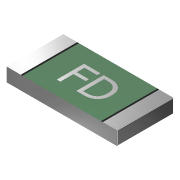
# Autodesk Inventor part: fuse
Saved by Autodesk Inventor 2012 (Build 160160000, 160)
## iProperties
Created: 2015-04-13
Part Number: fuse
Material: Default
Document SubType Name: Modeling
Designer: s42851
Density: 1 g/cm^3
Author: s42851
Autodesk Inventor part; units mm, degrees
ref_plane "YZ Plane" through (0, 0, 0) normal (1, 0, 0) x (0, 1, 0)
ref_plane "XZ Plane" through (0, 0, 0) normal (0, 1, 0) x (-1, 0, 0)
ref_plane "XY Plane" through (0, 0, 0) normal (0, 0, 1) x (1, 0, 0)
sketch "Sketch1" plane through (0, 0, 0) normal (0, 0, 1) x (1, 0, 0)
  line L0 (0, 0) -> (3.25, 0)
  line L1 (3.25, 0) -> (3.25, 1.65)
  line L2 (3.25, 1.65) -> (0, 1.65)
  line L3 (0, 1.65) -> (0, 0)
  dimension "d0" = 1.65
  dimension "d1" = 3.25
  constraints: 8 end point, 2 parallel, 1 horizontal, 1 perpendicular
  measures "d0" distance of L2.end L0.start
  measures "d1" distance of L0.start L0.end
extrude "Extrusion1" add sketch "Sketch1" along normal blind 0.4
sketch "Sketch2" plane through (0, 0, 0.4) normal (0, 0, 1) x (1, 0, 0)
  line L0 (0, 0) -> (0, 1.65) projected
  line L1 (3.25, 0) -> (0, 0) projected
  line L2 (0, 1.65) -> (3.25, 1.65) projected
  line L3 (0.425, 1.65) -> (0.425, 0)
  line L4 (0.475, 1.65) -> (0.475, 0)
  line L5 (0.425, 1.65) -> (0.475, 1.65)
  line L6 (0.425, 0) -> (0.475, 0)
  dimension "d4" = 0.425
  dimension "d7" = 0.05
  constraints: 8 end point, 2 parallel, 2 point on line, 1 collinear, 1 perpendicular
  measures "d4" distance between parallel lines of L0 L3
  measures "d7" distance between parallel lines of L3 L4
extrude "Extrusion2" cut sketch "Sketch2" against normal blind 0.001 contours L3 L2 L4 L1
ref_plane "Work Plane1" through (1.625, 0, 0) normal (1, 0, 0) x (0, 0, -1)
mirror "Mirror1" about plane through (1.625, 0, 0) normal (1, 0, 0) of "Extrusion2"
sketch "Sketch3" plane through (0, 0, 0.4) normal (0, 0, 1) x (1, 0, 0)
  line L0 (0.9936, 1.2023) -> (2.3385, 1.2023) construction
  line L1 (2.3385, 1.2023) -> (2.3385, 0.3392) construction
  line L2 (2.3385, 0.3392) -> (0.9936, 0.3392) construction
  line L3 (0.9936, 0.3392) -> (0.9936, 1.2023) construction
  line L4 (1.553, 1.1076) -> (1.1809, 1.1076)
  line L5 (1.1809, 1.1076) -> (1.1809, 0.882)
  line L6 (1.1809, 0.882) -> (1.5375, 0.882)
  line L7 (1.5375, 0.882) -> (1.5375, 0.7874)
  line L8 (1.5375, 0.7874) -> (1.1809, 0.7874)
  line L9 (1.1809, 0.7874) -> (1.1809, 0.4023)
  line L10 (1.1809, 0.4023) -> (1.0746, 0.4023)
  line L11 (1.0746, 0.4023) -> (1.0746, 1.2023)
  line L12 (1.0746, 1.2023) -> (1.553, 1.2023)
  line L13 (1.553, 1.2023) -> (1.553, 1.1076)
  spline S0 degree 2 poles (2.2791, 0.8016) (2.2791, 0.6921) (2.1903, 0.5157) (2.1158, 0.4665) knots 0 0 0 1 2 2 2
  spline S1 degree 2 poles (2.1158, 0.4665) (2.0548, 0.4282) (1.9297, 0.4023) (1.8325, 0.4023) knots 0 0 0 1 2 2 2
  line L14 (1.8325, 0.4023) -> (1.6483, 0.4023)
  line L15 (1.6483, 0.4023) -> (1.6483, 1.2023)
  line L16 (1.6483, 1.2023) -> (1.8305, 1.2023)
  spline S2 degree 2 poles (1.8305, 1.2023) (1.9433, 1.2023) (2.0717, 1.1686) (2.1171, 1.1387) knots 0 0 0 1 2 2 2
  spline S3 degree 2 poles (2.1171, 1.1387) (2.1942, 1.0875) (2.2791, 0.9183) (2.2791, 0.8016) knots 0 0 0 1 2 2 2
  spline S4 degree 2 poles (2.1683, 0.8029) (2.1683, 0.895) (2.1073, 1.0253) (2.047, 1.0622) knots 0 0 0 1 2 2 2
  spline S5 degree 2 poles (2.047, 1.0622) (2.0043, 1.0875) (1.9077, 1.1102) (1.8357, 1.1102) knots 0 0 0 1 2 2 2
  line L17 (1.8357, 1.1102) -> (1.7547, 1.1102)
  line L18 (1.7547, 1.1102) -> (1.7547, 0.4943)
  line L19 (1.7547, 0.4943) -> (1.8357, 0.4943)
  spline S6 degree 2 poles (1.8357, 0.4943) (1.9064, 0.4943) (2.0133, 0.517) (2.0568, 0.5475) knots 0 0 0 1 2 2 2
  spline S7 degree 2 poles (2.0568, 0.5475) (2.1125, 0.5851) (2.1683, 0.7096) (2.1683, 0.8029) knots 0 0 0 1 2 2 2
  point P0 (0, 0)
  constraints: 2 other
fillet "Fillet1" radius 0.02 8 edges at (3.25, 0.825, 0.4) (3.25, 0, 0.2) (3.25, 0.825, 0) (3.25, 1.65, 0.2) (0, 0.825, 0.4) (0, 1.65, 0.2) (0, 0.825, 0) (0, 0, 0.2)
extrude "Extrusion3" add sketch "Sketch3" along normal blind 0.001
body "Solid1"
